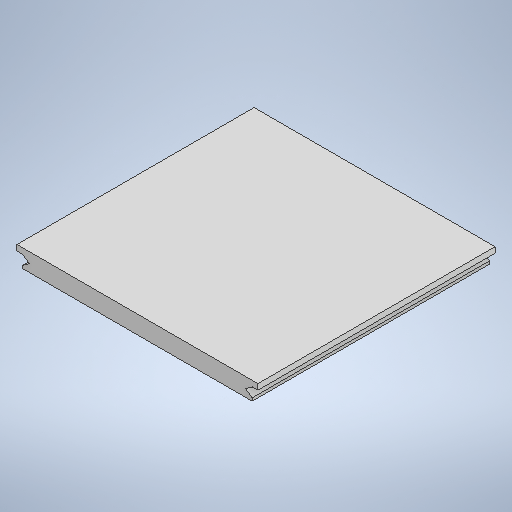
# Autodesk Inventor part: channel_lid
Saved by Autodesk Inventor 2025 (Build 290162000, 162)
## iProperties
Created: 2024-08-08
Part Number: channel_lid
Material: Generic
Document SubType Name: Modeling
Designer: ethan
Density: 1 g/cm^3
Appearance: Default
Author: ethan
Autodesk Inventor part; units mm, degrees
ref_plane "YZ Plane" through (0, 0, 0) normal (1, 0, 0) x (0, 1, 0)
ref_plane "XZ Plane" through (0, 0, 0) normal (0, 1, 0) x (-1, 0, 0)
ref_plane "XY Plane" through (0, 0, 0) normal (0, 0, 1) x (1, 0, 0)
sketch "Sketch1" plane through (0, 0, 0) normal (0, 0, 1) x (1, 0, 0)
  line L0 (50.8, 0) -> (50.8, 1.2)
  line L1 (50.8, 1.2) -> (0, 1.2)
  line L2 (0, 1.2) -> (0, 0)
  line L3 (0, 0) -> (1.2, 0) construction
  line L4 (1.2, 0) -> (1.2, -7.6054) construction
  line L5 (1.2, -7.6054) -> (0, -7.6054) construction
  line L6 (0, -7.6054) -> (0, 0) construction
  line L7 (50.8, 0) -> (49.6, 0) construction
  line L8 (49.6, 0) -> (49.6, -9.5013) construction
  line L9 (49.6, -9.5013) -> (50.8, -9.5013) construction
  line L10 (50.8, -9.5013) -> (50.8, 0) construction
  line L11 (1.2, 0) -> (1.2, -2) construction
  line L12 (1.2, -1) -> (2.614, -1) construction
  line L13 (1.2, -2) -> (2.614, -1)
  line L14 (1.2, 0) -> (2.614, -1)
  line L15 (1.2, -2) -> (1.2, -2.6)
  line L16 (1.2, -2.6) -> (49.6, -2.6)
  line L17 (49.6, -2.6) -> (49.6, -2)
  line L18 (49.6, -2) -> (49.6, 0) construction
  line L19 (49.6, -1) -> (48.186, -1) construction
  line L20 (49.6, -2) -> (48.186, -1)
  line L21 (49.6, 0) -> (48.186, -1)
  line L22 (0, 0) -> (1.2, 0)
  line L23 (49.6, 0) -> (50.8, 0)
  dimension "Width" = 50.8
  dimension "Thickness" = 1.2
  dimension "Leftwall" = 1.2
  dimension "Rightwall" = 1.2
  dimension "LTheight" = 2
  dimension "LTwidth" = 1.414
  dimension "BThickness" = 0.6
  dimension "BThicknessR" = 0.6
  dimension "RTWidth" = 1.414
  constraints: 48 end point, 7 parallel, 6 horizontal, 5 perpendicular, 4 point on line, 2 midpoint, 1 vertical
  measures "Width" distance of L1.end L0.end
  measures "Thickness" distance of L0.end L0.start
  measures "Leftwall" distance of L4.end L5.end
  measures "Rightwall" distance of L9.end L8.end
  measures "LTheight" distance of L3.end L11.end
  measures "LTwidth" distance of L12.start L12.end
  measures "BThickness" distance of L11.end L15.end
  measures "BThicknessR" distance of L16.end L17.end
  measures "RTWidth" distance of L19.start L19.end
extrude "Extrusion1" add sketch "Sketch1" along normal blind 50
equation "\"Rightwall\" = Leftwall"
equation "\"BThicknessR\" = BThickness"
equation "\"RTWidth\" = LTwidth"
body "Solid1"
